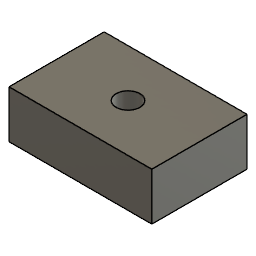
manual_box_hole (Autodesk Fusion 360 design; units mm, degrees)
Autodesk Fusion 360 part; units mm, degrees
sketch "草图1" plane through (0, 0, 0) normal (0, 1, 0) x (1, 0, 0)
  line L0 (0, 0) -> (60, 0)
  line L1 (60, 0) -> (60, 40)
  line L2 (60, 40) -> (0, 40)
  line L3 (0, 40) -> (0, 0)
  constraint horizontal L0
  constraint vertical L1
  constraint horizontal L2
  constraint vertical L3
  constraint coincident L0.start L3.end
extrude "拉伸1" add sketch "草图1" along normal blind 20
sketch "草图2" plane through (0, 20, 0) normal (0, 1, 0) x (-1, 0, 0)
  line L0 (0, -40) -> (0, 0)
  line L1 (0, 0) -> (-60, 0)
  line L2 (-60, 0) -> (-60, -40)
  line L3 (-60, -40) -> (0, -40)
  line L4 (0, 0) -> (-60, -40) construction
  line L5 (0, -40) -> (-60, 0) construction
  circle A0 centre (-30, -20) radius 5
  dimension "d3" = 10
  constraint coincident L0.end L1.start
  constraint coincident L2.end L3.start
  constraint coincident L0.start L3.end
  constraint coincident L1.end L2.start
  constraint midpoint L4 A0.centre
  measures "d3" diameter of A0
extrude "拉伸2" cut sketch "草图2" against normal through all contours A0
